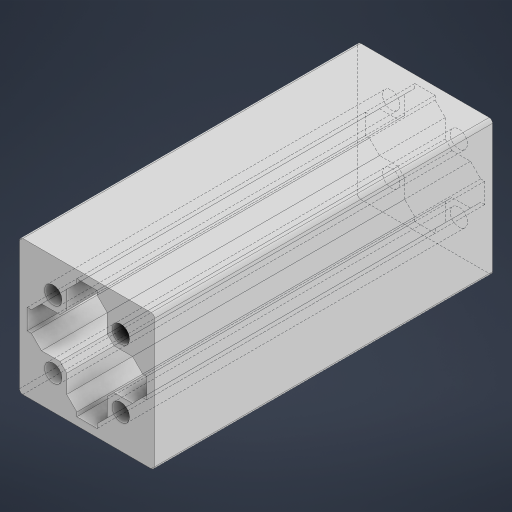
# Autodesk Inventor part: 100100W-PROFILE
Saved by Autodesk Inventor 2023 (Build 270158000, 158)
## iProperties
Created: 2025-09-03
Part Number: 100100W-PROFILE
Material: 일반
Document SubType Name: Modeling
Designer: k
Density: 1 g/cm^3
Appearance: 기본값
Author: k
Autodesk Inventor part; units mm, degrees
ref_plane "YZ Plane" through (0, 0, 0) normal (1, 0, 0) x (0, 1, 0)
ref_plane "XZ Plane" through (0, 0, 0) normal (0, 1, 0) x (-1, 0, 0)
ref_plane "XY Plane" through (0, 0, 0) normal (0, 0, 1) x (1, 0, 0)
sketch "스케치1" plane through (0, 0, 0) normal (0, 0, 1) x (1, 0, 0)
  line L0 (97.2793, -16.1712) -> (97.2793, -63.6712)
  line L1 (99.7793, -13.6712) -> (147.2793, -13.6712)
  circle A0 centre (122.2793, -38.6712) radius 6.5
  line L2 (139.7793, -19.4712) -> (147.2793, -19.4712)
  line L3 (127.2775, -48.6712) -> (132.2793, -43.6694)
  line L4 (127.2775, -48.6712) -> (113.6148, -48.6712)
  line L5 (132.2793, -30.0067) -> (132.2793, -43.6694)
  line L6 (139.7793, -22.5067) -> (132.2793, -30.0067)
  line L7 (139.7793, -19.4712) -> (139.7793, -22.5067)
  line L8 (103.0793, -56.1712) -> (103.0793, -63.6712)
  line L9 (106.1148, -56.1712) -> (113.6148, -48.6712)
  line L10 (103.0793, -56.1712) -> (106.1148, -56.1712)
  arc A1 (99.7793, -13.6712) -> (97.2793, -16.1712) centre (99.7793, -16.1712) ccw
  line L11 (197.2793, -16.1712) -> (197.2793, -63.6712)
  line L12 (194.7793, -13.6712) -> (147.2793, -13.6712)
  circle A2 centre (172.2793, -38.6712) radius 6.5
  line L13 (154.7793, -19.4712) -> (147.2793, -19.4712)
  line L14 (167.281, -48.6712) -> (162.2793, -43.6694)
  line L15 (167.281, -48.6712) -> (180.9437, -48.6712)
  line L16 (162.2793, -30.0067) -> (162.2793, -43.6694)
  line L17 (154.7793, -22.5067) -> (162.2793, -30.0067)
  line L18 (154.7793, -19.4712) -> (154.7793, -22.5067)
  line L19 (191.4793, -56.1712) -> (191.4793, -63.6712)
  line L20 (191.4793, -56.1712) -> (188.4437, -56.1712)
  line L21 (188.4437, -56.1712) -> (180.9437, -48.6712)
  arc A3 (197.2793, -16.1712) -> (194.7793, -13.6712) centre (194.7793, -16.1712) ccw
  line L22 (97.2793, -111.1712) -> (97.2793, -63.6712)
  line L23 (99.7793, -113.6712) -> (147.2793, -113.6712)
  circle A4 centre (122.2793, -88.6712) radius 6.5
  line L24 (139.7793, -107.8712) -> (147.2793, -107.8712)
  line L25 (127.2775, -78.6712) -> (132.2793, -83.6729)
  line L26 (127.2775, -78.6712) -> (113.6148, -78.6712)
  line L27 (132.2793, -97.3356) -> (132.2793, -83.6729)
  line L28 (139.7793, -104.8356) -> (132.2793, -97.3356)
  line L29 (139.7793, -107.8712) -> (139.7793, -104.8356)
  line L30 (103.0793, -71.1712) -> (103.0793, -63.6712)
  line L31 (103.0793, -71.1712) -> (106.1148, -71.1712)
  line L32 (106.1148, -71.1712) -> (113.6148, -78.6712)
  arc A5 (97.2793, -111.1712) -> (99.7793, -113.6712) centre (99.7793, -111.1712) ccw
  line L33 (154.7793, -104.8356) -> (162.2793, -97.3356)
  line L34 (162.2793, -97.3356) -> (162.2793, -83.6729)
  line L35 (167.281, -78.6712) -> (162.2793, -83.6729)
  circle A6 centre (172.2793, -88.6712) radius 6.5
  line L36 (167.281, -78.6712) -> (180.9437, -78.6712)
  line L37 (188.4437, -71.1712) -> (180.9437, -78.6712)
  line L38 (191.4793, -71.1712) -> (188.4437, -71.1712)
  line L39 (191.4793, -71.1712) -> (191.4793, -63.6712)
  line L40 (197.2793, -111.1712) -> (197.2793, -63.6712)
  arc A7 (194.7793, -113.6712) -> (197.2793, -111.1712) centre (194.7793, -111.1712) ccw
  line L41 (154.7793, -107.8712) -> (154.7793, -104.8356)
  line L42 (194.7793, -113.6712) -> (147.2793, -113.6712)
  line L43 (154.7793, -107.8712) -> (147.2793, -107.8712)
  point P0 (97.2793, -13.6712)
  point P1 (169.3645, -19.4712)
  point P2 (197.2793, -13.6712)
  point P3 (97.2793, -113.6712)
  point P4 (197.2793, -113.6712)
  dimension "d11" = 50
  dimension "d12" = 50
  dimension "d15" = 13
  dimension "d18" = 5.8
  dimension "d21" = 2.5
  constraints: 88 end point, 8 centre point, 8 point on circle, 8 point on line, 3 vertical, 2 tangent, 1 horizontal
  measures "d11" distance of point (97.279, -13.671) L1.end
  measures "d12" distance of point (97.279, -13.671) L0.end
  measures "d15" diameter of A0
  measures "d18" distance between parallel lines of L1 L2
  measures "d21" radius of A1
extrude "돌출1" add sketch "스케치1" along normal blind 250
